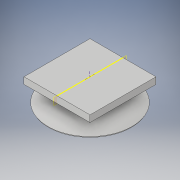
# Autodesk Inventor part: antenna
Saved by Autodesk Inventor 2019.1 (Build 231200000, 200)
## iProperties
Created: 2018-12-21
Part Number: antenna
Material: 一般
Document SubType Name: Modeling
Designer: Masaya
Density: 1 g/cm^3
Appearance: 既定
Author: Masaya
Autodesk Inventor part; units mm, degrees
ref_plane "YZ Plane" through (0, 0, 0) normal (1, 0, 0) x (0, 1, 0)
ref_plane "XZ Plane" through (0, 0, 0) normal (0, 1, 0) x (-1, 0, 0)
ref_plane "XY Plane" through (0, 0, 0) normal (0, 0, 1) x (1, 0, 0)
sketch "スケッチ1" plane through (0, 0, 0) normal (0, 1, 0) x (-1, 0, 0)
  line L0 (1000, 1000) -> (0, 1000)
  line L1 (0, 1000) -> (0, 0)
  line L2 (0, 0) -> (1000, 0)
  line L3 (1000, 0) -> (1000, 1000)
  dimension "d0" = 1000
  dimension "d1" = 1000
  constraints: 8 end point, 2 parallel, 1 coincident, 1 horizontal, 1 perpendicular
  measures "d0" distance of L0.start L0.end
  measures "d1" distance of L0.end L1.end
extrude "押し出し1" add sketch "スケッチ1" along normal blind 100
ref_plane "作業平面1" through (-500, 0, 1000) normal (1, 0, 0) x (0, 0, -1)
sketch "スケッチ3" plane through (-500, 0, 1000) normal (1, 0, 0) x (0, 0, -1)
  line L0 (0, 100) -> (1000, 100) projected
  point P0 (1000, 0)
  point P1 (500, 100)
  constraints: 1 midpoint
sketch "スケッチ4" plane through (-500, 0, 1000) normal (1, 0, 0) x (0, 0, -1)
  line L0 (0, 0) -> (1000, 0) projected
  arc A0 (1135.9702, -234.8449) -> (500, 0) centre (500, -978.5401) ccw
  arc A1 (1126.1954, -252.4708) -> (500, 0) centre (469.6535, -978.0695) ccw
  line L1 (1126.1954, -252.4708) -> (1135.9702, -234.8449)
  line L2 (500, 0) -> (500, -928.3168)
  constraints: 4 end point, 4 point on circle, 2 centre point, 1 midpoint, 1 vertical
revolve "回転1" add sketch "スケッチ4" angle 360 about axis through (-500, 0, 500) along (0, -1, 0)
